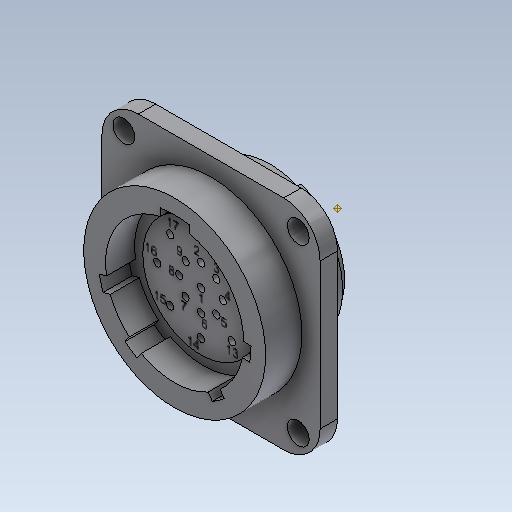
# Autodesk Inventor part: 360124
Saved by Autodesk Inventor 2020.1 (Build 241239000, 239)
## iProperties
GlobalPropertyList: <PropertyList/>
Part Number: 360124
Document SubType Name: Modeling
Created: 2003-10-08
Designer: Autodesk
Manufacturer: Standard
Standards Organization: Custom
Project: AIP
Description: AMP 3
Density: 1 g/cm^3
Categories: <MemberInstance><Categories><Category DisplayName="" Mnemonic="CABLEANDHARNESS" InternalName="e4a7e005-5e42-4d16-b293-125e7f0d0512"><Category DisplayName="" Mnemonic="CONNECTORS" InternalName="6f634eba-a678-4820-a31d-2c2d5ee6728e"><CategoryParameter DisplayName="" Mnemonic="REFDES" InternalName="c3740e8c-60ab-4d5d-8584-52b73222f2f0"/><Category DisplayName="" Mnemonic="DISCRETEWIRE" InternalName="9a3407de-09b2-4cdb-8c40-9708d5144a28"/></Category></Category></Categories><FamilyTemplate><FamilyTemplateParameters></FamilyTemplateParameters></FamilyTemplate><CategoryParameterMap><ParamToTemplateMap><ParamToTemplate CategoryParameter="//CategoryParameter[@InternalName='c3740e8c-60ab-4d5d-8584-52b73222f2f0']" ConstantValue=""/></ParamToTemplateMap></CategoryParameterMap></MemberInstance>
Material: Generic
Appearance: Aluminum - Flat
Company: Autodesk
Control State: 0
Master: False
Checked Out: False
Shininess: 64.0
Length Units: 11269
Angle Units: 11279
Time Units: 11290
Mass Units: 11286
Length Display Precision: 3
Angle Display Precision: 2
Compacted: True
Density: 0.0
Volumn: 0.0
Area: 0.0
PropertySet Name: Model Information
Subject: AMP 3
Author: Autodesk
Revision Number: 0
Autodesk Inventor part; units mm, degrees
ref_plane "YZ Plane" through (0, 0, 0) normal (1, 0, 0) x (0, 1, 0)
ref_plane "XZ Plane" through (0, 0, 0) normal (0, 1, 0) x (-1, 0, 0)
ref_plane "XY Plane" through (0, 0, 0) normal (0, 0, 1) x (1, 0, 0)
sketch "Sketch1" plane through (0, 0, 0) normal (0, 0, 1) x (1, 0, 0)
  line L0 (15, 15) -> (-15, 15)
  line L1 (-15, 15) -> (-15, -15)
  line L2 (-15, -15) -> (15, -15)
  line L3 (15, -15) -> (15, 15)
  point P0 (0, 0)
  point P1 (15, 0)
  point P2 (0, 15)
  dimension "d0" = 30
  constraints: 8 end point, 2 midpoint, 2 parallel, 2 perpendicular, 1 horizontal, 1 horizontal alignment, 1 vertical alignment
  measures "d0" distance of L0.start L0.end
extrude "Extrusion1" add sketch "Sketch1" along normal blind 2.3876
fillet "Fillet1" radius 5 4 edges at (15, 15, 1.1938) (-15, 15, 1.1938) (-15, -15, 1.1938) (15, -15, 1.1938)
sketch "Sketch2" plane through (0, 0, 2.3876) normal (0, 0, 1) x (1, 0, 0)
  line L0 (10, -15) -> (-10, -15) projected
  line L1 (15, 10) -> (15, -10) projected
  line L2 (-10, 15) -> (10, 15) projected
  line L3 (-15, -10) -> (-15, 10) projected
  point P0 (-12, 12)
  point P1 (12, 12)
  point P2 (12, -12)
  point P3 (-12, -12)
  dimension "d4" = 3
  dimension "d5" = 3
  dimension "d6" = 3
  dimension "d7" = 3
  constraints: 2 horizontal alignment, 2 vertical alignment
  measures "d4" distance from line of L3 point (-12, 12)
  measures "d5" distance from line of L2 point (-12, 12)
  measures "d6" distance from line of L0 point (-12, -12)
  measures "d7" distance from line of L1 point (12, -12)
hole "Hole1" at (-12, 12, 2.3876) at (12, 12, 2.3876) at (12, -12, 2.3876) at (-12, -12, 2.3876) direction (0, 0, -1) diameter 3 end through all
sketch "Sketch3" plane through (0, 0, 2.3876) normal (0, 0, 1) x (1, 0, 0)
  line L0 (15, 10) -> (15, -10) projected
  line L1 (-10, 15) -> (10, 15) projected
  circle A0 centre (0, 0) radius 12.5
  point P0 (15, 0)
  point P1 (0, 15)
  dimension "d15" = 25
  constraints: 2 midpoint, 1 centre point, 1 horizontal alignment, 1 vertical alignment
  measures "d15" diameter of A0
extrude "Extrusion2" add sketch "Sketch3" along normal blind 5
sketch "Sketch4" plane through (0, 0, 7.3876) normal (0, 0, 1) x (1, 0, 0)
  circle A0 centre (0, 0) radius 12.5 projected
  circle A1 centre (0, 0) radius 9.5
  dimension "d86" = 3
  constraints: 1 centre point, 1 coincident
  measures "d86" radial gap between concentric circles of A1 A0
extrude "Extrusion3" cut sketch "Sketch4" against normal blind 4 contours A1
sketch "Sketch5" plane through (0, 0, 7.3876) normal (0, 0, 1) x (1, 0, 0)
  circle A0 centre (0, 0) radius 9.5 projected
  circle A1 centre (0, 0) radius 12.5 projected
  circle A2 centre (0, 0) radius 10.5
  line L0 (-2, 9.2871) -> (-2, 10.3078)
  line L1 (2, 9.2871) -> (2, 10.3078)
  dimension "d23" = 4
  dimension "d85" = 2
  constraints: 4 end point, 4 point on circle, 2 parallel, 1 centre point, 1 coincident, 1 vertical
  measures "d23" distance between parallel lines of L1 L0
  measures "d85" radial gap between concentric circles of A1 A2
extrude "Extrusion4" cut sketch "Sketch5" against normal up to surface (4 mm away) contours A0 L0 A2 L1 picked at (-1.557, 9.6904)
sketch "Sketch6" plane through (0, 0, 7.3876) normal (0, 0, 1) x (1, 0, 0)
  line L0 (2, 10.3078) -> (2, 9.2871) projected
  arc A0 (-2, 9.2871) -> (2, 9.2871) centre (0, 0) ccw projected
  line L1 (-2, 9.2871) -> (-2, 10.3078) projected
  arc A1 (2, 10.3078) -> (-2, 10.3078) centre (0, 0) ccw projected
  circle A2 centre (0, 0) radius 12.5 projected
  circle A3 centre (0, 0) radius 10.5
  line L2 (-9.3841, -1.4792) -> (-10.3549, -1.7393)
  line L3 (-8.8665, -3.411) -> (-9.8373, -3.6712)
  line L4 (-6.2379, -7.1651) -> (-6.8143, -7.9884)
  line L5 (-5.176, -9.1356) -> (-4.5996, -8.3123)
  line L6 (4.5996, -8.3123) -> (5.176, -9.1356)
  line L7 (6.2379, -7.1651) -> (6.8143, -7.9884)
  line L8 (9.4984, 0.1728) -> (10.4997, 0.0852)
  line L9 (9.3241, -1.8196) -> (10.3253, -1.9072)
  dimension "d26" = 105
  dimension "d27" = 2
  dimension "d30" = 2
  dimension "d31" = 40
  dimension "d32" = 70
  dimension "d33" = 2
  dimension "d34" = 2
  dimension "d35" = 50
  constraints: 16 end point, 8 parallel, 1 coincident, 21 other
  measures "d26" angle of L1 L2
  measures "d27" distance between parallel lines of L3 L2
  measures "d30" distance between parallel lines of L5 L4
  measures "d31" angle of L3 L4
  measures "d32" angle of L6 L5
  measures "d33" distance between parallel lines of L7 L6
  measures "d34" distance between parallel lines of L8 L9
  measures "d35" angle of L9 L7
extrude "Extrusion5" cut sketch "Sketch6" against normal up to surface (4 mm away) contours L0 A0 L1 A1 | A3 L9 A0 L8 | L2 A0 L3 A3 | L7 A3 L6 A0 | L4 A0 L5 A3
sketch "Sketch7" plane through (0, 0, 3.3876) normal (0, 0, 1) x (1, 0, 0)
  arc A0 (2, 10.3078) -> (-2, 10.3078) centre (0, 0) ccw projected
  circle A1 centre (0, 0) radius 8
  arc A2 (-2, 9.2871) -> (-9.3841, -1.4792) centre (0, 0) ccw projected
  dimension "d84" = 1.5
  constraints: 1 centre point, 1 coincident
  measures "d84" radial gap between concentric circles of A2 A1
extrude "Extrusion6" add sketch "Sketch7" along normal blind 0.381
sketch "Sketch8" plane through (0, 0, 0) normal (0, 0, -1) x (-1, 0, 0)
  line L0 (-10, 15) -> (10, 15) projected
  line L1 (-15, -10) -> (-15, 10) projected
  circle A0 centre (0, 0) radius 10
  point P0 (-15, 0)
  point P1 (0, 15)
  dimension "d39" = 20
  constraints: 2 midpoint, 1 centre point, 1 horizontal alignment, 1 vertical alignment
  measures "d39" diameter of A0
extrude "Extrusion7" add sketch "Sketch8" along normal blind 5.715
sketch "Sketch9" plane through (0, 0, -5.715) normal (0, 0, -1) x (-1, 0, 0)
  circle A0 centre (0, 0) radius 10 projected
  circle A1 centre (0, 0) radius 9
  dimension "d83" = 1
  constraints: 1 centre point, 1 coincident
  measures "d83" radial gap between concentric circles of A0 A1
extrude "Extrusion8" add sketch "Sketch9" along normal blind 1.27 contours A1
sketch "Sketch10" plane through (0, 0, -6.985) normal (0, 0, -1) x (-1, 0, 0)
  circle A0 centre (0, 0) radius 9 projected
  circle A1 centre (0, 0) radius 8
  line L0 (-3, 7.4162) -> (-3, 8.4853)
  line L1 (3, 7.4162) -> (3, 8.4853)
  dimension "d46" = 6
  dimension "d82" = 1
  constraints: 4 end point, 4 point on circle, 2 parallel, 1 centre point, 1 coincident, 1 vertical
  measures "d46" distance between parallel lines of L1 L0
  measures "d82" radial gap between concentric circles of A1 A0
extrude "Extrusion9" cut sketch "Sketch10" against normal up to surface (1.27 mm away) contours L1 A1 L0 A0 picked at (-1.8485, 8.4268)
sketch "Sketch11" plane through (0, 0, 3.7686) normal (0, 0, 1) x (1, 0, 0)
  circle A0 centre (0, 0) radius 8 projected
  line L0 (0, 0) -> (0, 6) construction
  point P0 (0, 3)
  point P1 (-2.1213, 2.1213)
  point P2 (-3, 0)
  point P3 (-2.1213, -2.1213)
  point P4 (0, -3)
  point P5 (2.1213, -2.1213)
  point P6 (3, 0)
  point P7 (2.1213, 2.1213)
  point P8 (4.2426, 4.2426)
  point P9 (6, 0)
  point P10 (4.2426, -4.2426)
  point P11 (0, -6)
  point P12 (-4.2426, -4.2426)
  point P13 (-6, 0)
  point P14 (-4.2426, 4.2426)
  dimension "d49" = 3
  dimension "d52" = 360
  dimension "d87" = 6
  dimension "d90" = 360
  constraints: 2 coincident, 2 end point, 1 vertical, 1 vertical alignment, 18 other
  measures "d49" distance of point (0, 3) L0.start
  measures "d87" distance of L0.start L0.end
hole "Hole2" at (0, 0, 3.7686) at (0, 3, 3.7686) at (-2.1213, 2.1213, 3.7686) at (-3, 0, 3.7686) at (-2.1213, -2.1213, 3.7686) at (0, -3, 3.7686) at (2.1213, -2.1213, 3.7686) at (3, 0, 3.7686) at (2.1213, 2.1213, 3.7686) at (0, 6, 3.7686) at (4.2426, 4.2426, 3.7686) at (6, 0, 3.7686) at (4.2426, -4.2426, 3.7686) at (0, -6, 3.7686) at (-4.2426, -4.2426, 3.7686) at (-6, 0, 3.7686) at (-4.2426, 4.2426, 3.7686) direction (0, 0, -1) diameter 1 end through all
sketch "Sketch12" plane through (0, 0, -6.985) normal (0, 0, -1) x (-1, 0, 0)
  circle A0 centre (-3, 0) radius 0.5 projected
  circle A1 centre (0, -3) radius 0.5 projected
  circle A2 centre (3, 0) radius 0.5 projected
  circle A3 centre (0, 3) radius 0.5 projected
  circle A4 centre (0, 0) radius 0.5 projected
  circle A5 centre (2.1213, 2.1213) radius 0.5 projected
  circle A6 centre (2.1213, -2.1213) radius 0.5 projected
  circle A7 centre (-2.1213, -2.1213) radius 0.5 projected
  circle A8 centre (-2.1213, 2.1213) radius 0.5 projected
  point P0 (6, 0)
  point P1 (0, -6)
  point P2 (-6, 0)
  point P3 (0, 6)
  point P4 (-4.2426, 4.2426)
  point P5 (-4.2426, -4.2426)
  point P6 (4.2426, -4.2426)
  point P7 (4.2426, 4.2426)
  point P8 (0, 0)
  point P9 (0, 0)
hole "Hole3" at (0, 3, -6.985) at (2.1213, 2.1213, -6.985) at (3, 0, -6.985) at (2.1213, -2.1213, -6.985) at (0, 0, -6.985) at (-2.1213, 2.1213, -6.985) at (-3, 0, -6.985) at (-2.1213, -2.1213, -6.985) at (0, -3, -6.985) at (4.2426, 4.2426, -6.985) at (0, 6, -6.985) at (-4.2426, 4.2426, -6.985) at (-6, 0, -6.985) at (-4.2426, -4.2426, -6.985) at (0, -6, -6.985) at (4.2426, -4.2426, -6.985) at (6, 0, -6.985) direction (0, 0, 1) diameter 2 depth 9.5
sketch "Sketch13" plane through (0, 0, -6.985) normal (0, 0, -1) x (-1, 0, 0)
  arc A0 (-3, 8.4853) -> (3, 8.4853) centre (0, 0) ccw projected
  line L0 (3, 8.4853) -> (3, 7.4162) projected
  arc A1 (3, 7.4162) -> (-3, 7.4162) centre (0, 0) ccw projected
  circle A2 centre (0, 0) radius 8
  line L1 (-2.5, -8.6458) -> (-2.5, -7.5993)
  line L2 (2.5, -8.6458) -> (2.5, -7.5993)
  dimension "d68" = 5
  constraints: 5 point on circle, 4 end point, 3 parallel, 1 centre point, 1 coincident
  measures "d68" distance between parallel lines of L2 L1
extrude "Extrusion10" cut sketch "Sketch13" against normal up to surface (1.27 mm away) contours L1 A2 L2 A0
sketch "Sketch25" plane through (0, 0, 3.7686) normal (0, 0, 1) x (1, 0, 0)
  line L0 (-1.0163, 4.6819) -> (0.1279, 4.6819) construction
  line L1 (0.1279, 4.6819) -> (0.1279, 3.2031) construction
  line L2 (0.1279, 3.2031) -> (-1.0163, 3.2031) construction
  line L3 (-1.0163, 3.2031) -> (-1.0163, 4.6819) construction
  line L4 (3.2538, -0.055) -> (3.2538, 1.4238) construction
  line L5 (3.2538, 1.4238) -> (4.398, 1.4238) construction
  line L6 (4.398, 1.4238) -> (4.398, -0.055) construction
  line L7 (4.398, -0.055) -> (3.2538, -0.055) construction
  line L8 (1.6906, 2.4904) -> (1.6906, 3.9692) construction
  line L9 (1.6906, 3.9692) -> (2.8348, 3.9692) construction
  line L10 (2.8348, 3.9692) -> (2.8348, 2.4904) construction
  line L11 (2.8348, 2.4904) -> (1.6906, 2.4904) construction
  line L12 (-2.7944, -4.281) -> (-2.7944, -2.8021) construction
  line L13 (-2.7944, -2.8021) -> (-1.6502, -2.8021) construction
  line L14 (-1.6502, -2.8021) -> (-1.6502, -4.281) construction
  line L15 (-1.6502, -4.281) -> (-2.7944, -4.281) construction
  line L16 (-3.4049, 1.9851) -> (-3.4049, 3.4639) construction
  line L17 (-3.4049, 3.4639) -> (-2.2607, 3.4639) construction
  line L18 (-2.2607, 3.4639) -> (-2.2607, 1.9851) construction
  line L19 (-2.2607, 1.9851) -> (-3.4049, 1.9851) construction
  line L20 (-0.3938, -2.1662) -> (-0.3938, -0.6874) construction
  line L21 (-0.3938, -0.6874) -> (0.7504, -0.6874) construction
  line L22 (0.7504, -0.6874) -> (0.7504, -2.1662) construction
  line L23 (0.7504, -2.1662) -> (-0.3938, -2.1662) construction
  line L24 (0.0431, -4.9913) -> (0.0431, -3.5125) construction
  line L25 (0.0431, -3.5125) -> (1.1873, -3.5125) construction
  line L26 (1.1873, -3.5125) -> (1.1873, -4.9913) construction
  line L27 (1.1873, -4.9913) -> (0.0431, -4.9913) construction
  line L28 (-4.4721, -0.8803) -> (-4.4721, 0.5985) construction
  line L29 (-4.4721, 0.5985) -> (-3.3279, 0.5985) construction
  line L30 (-3.3279, 0.5985) -> (-3.3279, -0.8803) construction
  line L31 (-3.3279, -0.8803) -> (-4.4721, -0.8803) construction
  line L32 (-0.7955, 6.2805) -> (-0.7955, 7.7593) construction
  line L33 (-0.7955, 7.7593) -> (0.3487, 7.7593) construction
  line L34 (0.3487, 7.7593) -> (0.3487, 6.2805) construction
  line L35 (0.3487, 6.2805) -> (-0.7955, 6.2805) construction
  line L36 (2.6912, -3.4816) -> (2.6912, -2.0028) construction
  line L37 (2.6912, -2.0028) -> (3.8354, -2.0028) construction
  line L38 (3.8354, -2.0028) -> (3.8354, -3.4816) construction
  line L39 (3.8354, -3.4816) -> (2.6912, -3.4816) construction
  line L40 (6.0179, 0.2278) -> (6.0179, 1.7067) construction
  line L41 (6.0179, 1.7067) -> (7.1621, 1.7067) construction
  line L42 (7.1621, 1.7067) -> (7.1621, 0.2278) construction
  line L43 (7.1621, 0.2278) -> (6.0179, 0.2278) construction
  line L44 (3.4493, 4.5372) -> (3.4493, 6.016) construction
  line L45 (3.4493, 6.016) -> (4.5935, 6.016) construction
  line L46 (4.5935, 6.016) -> (4.5935, 4.5372) construction
  line L47 (4.5935, 4.5372) -> (3.4493, 4.5372) construction
  line L48 (3.4493, -6.362) -> (3.4493, -4.8831) construction
  line L49 (3.4493, -4.8831) -> (4.5935, -4.8831) construction
  line L50 (4.5935, -4.8831) -> (4.5935, -6.362) construction
  line L51 (4.5935, -6.362) -> (3.4493, -6.362) construction
  line L52 (-1.904, -8) -> (-1.904, -6.5212) construction
  line L53 (-1.904, -6.5212) -> (-0.7598, -6.5212) construction
  line L54 (-0.7598, -6.5212) -> (-0.7598, -8) construction
  line L55 (-0.7598, -8) -> (-1.904, -8) construction
  line L56 (-6.5, -4.8831) -> (-6.5, -3.4043) construction
  line L57 (-6.5, -3.4043) -> (-5.3558, -3.4043) construction
  line L58 (-5.3558, -3.4043) -> (-5.3558, -4.8831) construction
  line L59 (-5.3558, -4.8831) -> (-6.5, -4.8831) construction
  line L60 (-7.769, 0.2278) -> (-7.769, 1.7067) construction
  line L61 (-7.769, 1.7067) -> (-6.6248, 1.7067) construction
  line L62 (-6.6248, 1.7067) -> (-6.6248, 0.2278) construction
  line L63 (-6.6248, 0.2278) -> (-7.769, 0.2278) construction
  line L64 (-4.7426, 4.7426) -> (-4.7426, 6.2215) construction
  line L65 (-4.7426, 6.2215) -> (-3.5984, 6.2215) construction
  line L66 (-3.5984, 6.2215) -> (-3.5984, 4.7426) construction
  line L67 (-3.5984, 4.7426) -> (-4.7426, 4.7426) construction
  constraints: 34 other
ref_plane "Work Plane2" through (0, 0, -12.985) normal (0, 0, -1) x (-1, 0, 0)
ref_plane "Work Plane3" through (0, 0, -14.985) normal (0, 0, -1) x (-1, 0, 0)
equation "\"d5\" = d4"
equation "\"d6\" = d4"
equation "\"d7\" = d4"
equation "\"d30\" = d27"
equation "\"d33\" = d30"
equation "\"d34\" = d33"
body "Solid1"
